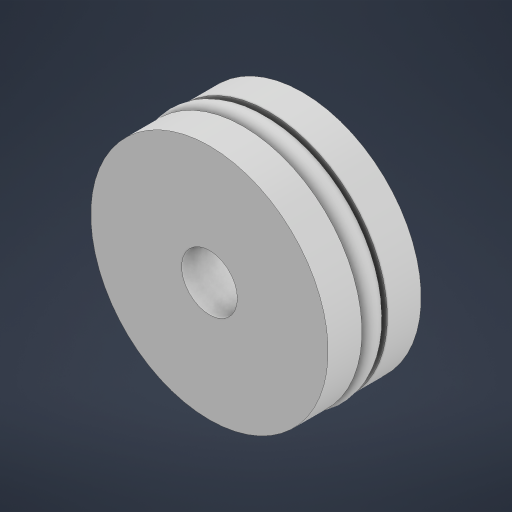
# Autodesk Inventor part: sf_Piston_1
Saved by Autodesk Inventor 2024 (Build 280153000, 153)
## iProperties
Created: 2024-03-20
Part Number: sf_Piston_1
Material: Generisch
Document SubType Name: Modeling
Designer: Simon
Density: 1 g/cm^3
Appearance: Vorgabe
Author: Simon
Autodesk Inventor part; units mm, degrees
ref_plane "YZ Plane" through (0, 0, 0) normal (1, 0, 0) x (0, 1, 0)
ref_plane "XZ Plane" through (0, 0, 0) normal (0, 1, 0) x (-1, 0, 0)
ref_plane "XY Plane" through (0, 0, 0) normal (0, 0, 1) x (1, 0, 0)
sketch "Skizze1" plane through (0, 0, 0) normal (1, 0, 0) x (0, 1, 0)
  line L0 (5.5, 14) -> (-5.5, 14)
  line L1 (-5.5, 14) -> (5.5, 14)
  line L2 (5.5, 14) -> (5.5, -0.0271)
  line L3 (5.5, -0.0271) -> (-5.5, -0.0271)
  line L4 (-5.5, -0.0271) -> (-5.5, 14)
  line L5 (0, -0.0271) -> (0, 14.2229)
  line L6 (0, -0.0271) -> (14.25, -0.0271) construction
  line L7 (-1.5, 11.223) -> (1.5, 11.223)
  line L8 (1.5, 11.223) -> (1.5, 14)
  line L9 (1.5, 14) -> (-1.5, 14)
  line L10 (-1.5, 14) -> (-1.5, 11.223)
  point P0 (0, 11.223)
  dimension "d0" = 11
  dimension "d2" = 14.25
  dimension "d3" = 90
  dimension "d4" = 3
  dimension "d5" = 4
  dimension "d6" = 4
  constraints: 22 end point, 4 parallel, 3 horizontal, 3 perpendicular, 2 point on line, 1 midpoint, 1 vertical
  measures "d0" distance of L0.end L0.start
  measures "d2" distance of L5.start L5.end
  measures "d3" angle of L6 L5
  measures "d4" distance of L9.end L8.end
  measures "d5" distance between parallel lines of L4 L10
  measures "d6" distance between parallel lines of L2 L8
revolve "Umdrehung1" add sketch "Skizze1" angle 360 about axis through (0, 5.5, -0.0271) along (0, -1, 0) contours L2 L3 L5 L7 L8 L0 | L3 L4 L0 L10 L7 L5
sketch "Skizze2" plane through (0, 0, 0) normal (1, 0, 0) x (0, 1, 0)
  line L0 (-1.5, 14) -> (-1.5, -14.0543) projected
  line L1 (1.5, 11.223) -> (-1.5, 11.223) projected
  line L2 (-1.5, 14) -> (1.5, 14)
  line L3 (1.5, 14) -> (1.5, 11.223)
  line L4 (1.5, 11.223) -> (-1.5, 11.223)
  line L5 (-1.5, 11.223) -> (-1.5, 14)
  circle A0 centre (0, 11.223) radius 1.5 construction
  circle A1 centre (0, 12.723) radius 1.5
  line L6 (6.3814, -0.0271) -> (7.4882, -0.0271) construction
  point P0 (0, 0)
  constraints: 10 end point, 2 horizontal, 2 parallel, 2 point on circle, 1 centre point, 1 midpoint, 1 perpendicular, 1 point on line, 1 vertical alignment, 2 other
revolve "Umdrehung2" add sketch "Skizze2" angle 360 about axis through (0, 6.3814, -0.0271) along (0, 1, 0) separate body contours A1 L2 | A1 L2
sketch "Skizze3" plane through (0, -5.5, -0.0271) normal (0, -1, 0) x (1, 0, 0)
  point P0 (0, 0.0271)
hole "Bohrung1" at (0, -5.5, 0) direction (0, 1, 0) diameter 6.6 depth 11 bodies 1 clearance for "Flachkopfsenkschraube ISO 2009/7046" size "M6" standard "ISO"
